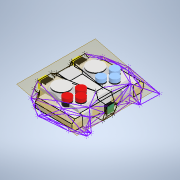
# Autodesk Inventor part: Obudowa_v1_srodek_2d
Saved by Autodesk Inventor 2020 (Build 240168000, 168)
## iProperties
Created: 2020-04-14
Part Number: Obudowa_v1_srodek_2d
Material: Generic
Document SubType Name: Modeling
Designer: atmat
Density: 1 g/cm^3
Appearance: Default
Author: atmat
Autodesk Inventor part; units mm, degrees
ref_plane "XY Plane" through (0, 0, 0) normal (0, 0, 1) x (1, 0, 0)
sketch "Sketch1" plane through (0, 0, 0) normal (0, 1, 0) x (-1, 0, 0)
  line L0 (35.245, 45.085) -> (-35.245, 45.085)
  line L1 (-35.245, 45.085) -> (-35.245, -45.085)
  line L2 (-35.245, -45.085) -> (35.245, -45.085)
  line L3 (35.245, -45.085) -> (35.245, 45.085)
  circle A0 centre (11.745, 29.845) radius 13
  circle A1 centre (11.745, -29.845) radius 13
  line L4 (-10.475, 45.085) -> (-10.475, -45.085) construction
  circle A2 centre (-10.475, 41.905) radius 6.5
  circle A3 centre (-10.475, 17.775) radius 6.5
  circle A4 centre (-10.475, -17.775) radius 6.5
  circle A5 centre (-10.475, -41.905) radius 6.5
  circle A6 centre (-22.545, 29.845) radius 6.5
  circle A7 centre (-22.545, -29.845) radius 6.5
  point P0 (0, 0)
  dimension "d58" = 70.49
  dimension "d0" = 90.17
  dimension "d1" = 45.085
  dimension "d2" = 35.245
  dimension "d3" = 70.49
  dimension "d4" = 15.24
  dimension "d5" = 15.24
  dimension "d6" = 23.5
  dimension "d7" = 23.5
  dimension "d8" = 26
  dimension "d9" = 26
  dimension "d10" = 45.72
  dimension "d11" = 13
  dimension "d12" = 13
  dimension "d13" = 13
  dimension "d14" = 13
  dimension "d15" = 3.18
  dimension "d16" = 3.18
  dimension "d17" = 24.13
  dimension "d18" = 24.13
  dimension "d19" = 13
  dimension "d20" = 12.07
  dimension "d21" = 12.07
  dimension "d22" = 0
  dimension "d23" = 0
  dimension "d24" = 13
  constraints: 10 end point, 8 centre point, 6 point on line, 2 parallel, 2 perpendicular, 1 horizontal
  measures "d0" distance of L2.end L0.start
  measures "d1" distance from line of point (0, 0) L0
  measures "d2" distance from line of point (0, 0) L3
  measures "d3" distance of L1.end L2.end
  measures "d4" distance from line of L0 A0.centre
  measures "d5" distance from line of L2 A1.centre
  measures "d6" distance from line of L3 A1.centre
  measures "d7" distance from line of L3 A0.centre
  measures "d8" diameter of A0
  measures "d9" diameter of A1
  measures "d10" distance between parallel lines of L3 L4
  measures "d11" diameter of A2
  measures "d12" diameter of A3
  measures "d13" diameter of A4
  measures "d14" diameter of A5
  measures "d15" distance from line of L0 A2.centre
  measures "d16" distance from line of L2 A5.centre
  measures "d17" distance of A3.centre A2.centre
  measures "d18" distance of A4.centre A5.centre
  measures "d19" diameter of A6
  measures "d20" horizontal distance of A2.centre A6.centre
  measures "d21" horizontal distance of A5.centre A7.centre
  measures "d22" vertical distance of A6.centre A0.centre
  measures "d23" vertical distance of A7.centre A1.centre
  measures "d24" diameter of A7
extrude "Extrusion1" add sketch "Sketch1" along normal blind 11 contours A0 | A1
sketch "Sketch2" plane through (0, 0, 0) normal (0, 1, 0) x (-1, 0, 0)
  line L0 (35.245, 45.085) -> (-35.245, 45.085)
  line L1 (-35.245, 45.085) -> (-35.245, -45.085)
  line L2 (-35.245, -45.085) -> (35.245, -45.085)
  line L3 (35.245, -45.085) -> (35.245, 45.085)
  circle A0 centre (11.745, 29.845) radius 13
  circle A1 centre (11.745, -29.845) radius 13
  line L4 (-10.475, 45.085) -> (-10.475, -45.085) construction
  circle A2 centre (-10.475, 41.905) radius 6.5
  circle A3 centre (-10.475, 17.775) radius 6.5
  circle A4 centre (-10.475, -17.775) radius 6.5
  circle A5 centre (-10.475, -41.905) radius 6.5
  circle A6 centre (-22.545, 29.845) radius 6.5
  circle A7 centre (-22.545, -29.845) radius 6.5
  point P0 (0, 0)
  dimension "d27" = 90.17
  dimension "d28" = 45.085
  dimension "d29" = 35.245
  dimension "d30" = 70.49
  dimension "d31" = 15.24
  dimension "d32" = 15.24
  dimension "d33" = 23.5
  dimension "d34" = 23.5
  dimension "d35" = 26
  dimension "d36" = 26
  dimension "d37" = 45.72
  dimension "d38" = 13
  dimension "d39" = 13
  dimension "d40" = 13
  dimension "d41" = 13
  dimension "d42" = 3.18
  dimension "d43" = 3.18
  dimension "d44" = 24.13
  dimension "d45" = 24.13
  dimension "d46" = 13
  dimension "d47" = 12.07
  dimension "d48" = 12.07
  dimension "d49" = 0
  dimension "d50" = 0
  dimension "d51" = 13
  constraints: 10 end point, 8 centre point, 6 point on line, 2 parallel, 2 perpendicular, 1 horizontal
  measures "d27" distance of L2.end L0.start
  measures "d28" distance from line of point (0, 0) L0
  measures "d29" distance from line of point (0, 0) L3
  measures "d30" distance of L1.end L2.end
  measures "d31" distance from line of L0 A0.centre
  measures "d32" distance from line of L2 A1.centre
  measures "d33" distance from line of L3 A1.centre
  measures "d34" distance from line of L3 A0.centre
  measures "d35" diameter of A0
  measures "d36" diameter of A1
  measures "d37" distance between parallel lines of L3 L4
  measures "d38" diameter of A2
  measures "d39" diameter of A3
  measures "d40" diameter of A4
  measures "d41" diameter of A5
  measures "d42" distance from line of L0 A2.centre
  measures "d43" distance from line of L2 A5.centre
  measures "d44" distance of A3.centre A2.centre
  measures "d45" distance of A4.centre A5.centre
  measures "d46" diameter of A6
  measures "d47" horizontal distance of A2.centre A6.centre
  measures "d48" horizontal distance of A5.centre A7.centre
  measures "d49" vertical distance of A6.centre A0.centre
  measures "d50" vertical distance of A7.centre A1.centre
  measures "d51" diameter of A7
extrude "Extrusion2" add sketch "Sketch2" along normal blind 7 contours A2 L0 | L0 A2 | A5 L2 | L2 A5 | A3 | A4 | A6 | A7
ref_plane "Work Plane1" through (0, 7, 0) normal (0, 1, 0) x (-1, 0, 0)
sketch "Sketch3" plane through (0, 7, 0) normal (0, 1, 0) x (-1, 0, 0)
  line L0 (35.245, 45.085) -> (-35.245, 45.085)
  line L1 (-35.245, 45.085) -> (-35.245, -45.085)
  line L2 (-35.245, -45.085) -> (35.245, -45.085)
  line L3 (35.245, -45.085) -> (35.245, 45.085)
  circle A0 centre (11.745, 29.845) radius 13
  circle A1 centre (11.745, -29.845) radius 13
  line L4 (-10.475, 45.085) -> (-10.475, -45.085) construction
  circle A2 centre (-10.475, 41.905) radius 6.5
  circle A3 centre (-10.475, 17.775) radius 6.5
  circle A4 centre (-10.475, -17.775) radius 6.5
  circle A5 centre (-10.475, -41.905) radius 6.5
  circle A6 centre (-22.545, 29.845) radius 6.5
  circle A7 centre (-22.545, -29.845) radius 6.5
  point P0 (0, 0)
  dimension "d55" = 90.17
  dimension "d56" = 45.085
  dimension "d57" = 35.245
  dimension "d58" = 70.49
  dimension "d59" = 15.24
  dimension "d60" = 15.24
  dimension "d61" = 23.5
  dimension "d62" = 23.5
  dimension "d63" = 26
  dimension "d64" = 26
  dimension "d65" = 45.72
  dimension "d66" = 13
  dimension "d67" = 13
  dimension "d68" = 13
  dimension "d69" = 13
  dimension "d70" = 3.18
  dimension "d71" = 3.18
  dimension "d72" = 24.13
  dimension "d73" = 24.13
  dimension "d74" = 13
  dimension "d75" = 12.07
  dimension "d76" = 12.07
  dimension "d77" = 0
  dimension "d78" = 0
  dimension "d79" = 13
  constraints: 10 end point, 8 centre point, 6 point on line, 2 parallel, 2 perpendicular, 1 horizontal
  measures "d55" distance of L2.end L0.start
  measures "d56" distance from line of point (0, 0) L0
  measures "d57" distance from line of point (0, 0) L3
  measures "d58" distance of L1.end L2.end
  measures "d59" distance from line of L0 A0.centre
  measures "d60" distance from line of L2 A1.centre
  measures "d61" distance from line of L3 A1.centre
  measures "d62" distance from line of L3 A0.centre
  measures "d63" diameter of A0
  measures "d64" diameter of A1
  measures "d65" distance between parallel lines of L3 L4
  measures "d66" diameter of A2
  measures "d67" diameter of A3
  measures "d68" diameter of A4
  measures "d69" diameter of A5
  measures "d70" distance from line of L0 A2.centre
  measures "d71" distance from line of L2 A5.centre
  measures "d72" distance of A3.centre A2.centre
  measures "d73" distance of A4.centre A5.centre
  measures "d74" diameter of A6
  measures "d75" horizontal distance of A2.centre A6.centre
  measures "d76" horizontal distance of A5.centre A7.centre
  measures "d77" vertical distance of A6.centre A0.centre
  measures "d78" vertical distance of A7.centre A1.centre
  measures "d79" diameter of A7
extrude "Extrusion3" add sketch "Sketch3" along normal blind 6 separate body contours A2 L0 | L0 A2 | A5 L2 | L2 A5 | A3 | A4 | A6 | A7
sketch "Sketch4" plane through (0, 0, 0) normal (0, 1, 0) x (-1, 0, 0)
  line L0 (35.245, 45.085) -> (-35.245, 45.085)
  line L1 (-35.245, 45.085) -> (-35.245, -45.085)
  line L2 (-35.245, -45.085) -> (35.245, -45.085)
  line L3 (35.245, -45.085) -> (35.245, 45.085)
  circle A0 centre (11.745, 29.845) radius 13
  circle A1 centre (11.745, -29.845) radius 13
  line L4 (-10.475, 45.085) -> (-10.475, -45.085) construction
  circle A2 centre (-10.475, 41.905) radius 6.5
  circle A3 centre (-10.475, 17.775) radius 6.5
  circle A4 centre (-10.475, -17.775) radius 6.5
  circle A5 centre (-10.475, -41.905) radius 6.5
  circle A6 centre (-22.545, 29.845) radius 6.5
  circle A7 centre (-22.545, -29.845) radius 6.5
  point P0 (0, 0)
  dimension "d82" = 90.17
  dimension "d83" = 45.085
  dimension "d84" = 35.245
  dimension "d85" = 70.49
  dimension "d86" = 15.24
  dimension "d87" = 15.24
  dimension "d88" = 23.5
  dimension "d89" = 23.5
  dimension "d90" = 26
  dimension "d91" = 26
  dimension "d92" = 45.72
  dimension "d93" = 13
  dimension "d94" = 13
  dimension "d95" = 13
  dimension "d96" = 13
  dimension "d97" = 3.18
  dimension "d98" = 3.18
  dimension "d99" = 24.13
  dimension "d100" = 24.13
  dimension "d101" = 13
  dimension "d102" = 12.07
  dimension "d103" = 12.07
  dimension "d104" = 0
  dimension "d105" = 0
  dimension "d106" = 13
  constraints: 10 end point, 8 centre point, 6 point on line, 2 parallel, 2 perpendicular, 1 horizontal
  measures "d82" distance of L2.end L0.start
  measures "d83" distance from line of point (0, 0) L0
  measures "d84" distance from line of point (0, 0) L3
  measures "d85" distance of L1.end L2.end
  measures "d86" distance from line of L0 A0.centre
  measures "d87" distance from line of L2 A1.centre
  measures "d88" distance from line of L3 A1.centre
  measures "d89" distance from line of L3 A0.centre
  measures "d90" diameter of A0
  measures "d91" diameter of A1
  measures "d92" distance between parallel lines of L3 L4
  measures "d93" diameter of A2
  measures "d94" diameter of A3
  measures "d95" diameter of A4
  measures "d96" diameter of A5
  measures "d97" distance from line of L0 A2.centre
  measures "d98" distance from line of L2 A5.centre
  measures "d99" distance of A3.centre A2.centre
  measures "d100" distance of A4.centre A5.centre
  measures "d101" diameter of A6
  measures "d102" horizontal distance of A2.centre A6.centre
  measures "d103" horizontal distance of A5.centre A7.centre
  measures "d104" vertical distance of A6.centre A0.centre
  measures "d105" vertical distance of A7.centre A1.centre
  measures "d106" diameter of A7
extrude "Extrusion4" add sketch "Sketch4" against normal blind 18 contours L3 L2 A5 L1 L0 A2 | A2 L0 | L2 A5 | A0 | A1 | A3 | A4 | A6 | A7 picked at (-10.0855, 41.5356) picked at (-10.2378, -41.8714) bodies 1
ref_plane "Work Plane2" through (-35.245, 0, 0) normal (1, 0, 0) x (0, 1, 0)
sketch "Sketch6" plane through (-35.245, 0, 0) normal (1, 0, 0) x (0, 1, 0)
  circle A0 centre (0, -29.845) radius 6.5
  circle A1 centre (0, 29.845) radius 6.5
  line L0 (0, -45.085) -> (0, 45.085) projected
  line L1 (6, -23.845) -> (-6, -23.845)
  line L2 (-6, -23.845) -> (-6, -35.845)
  line L3 (-6, -35.845) -> (6, -35.845)
  line L4 (6, -35.845) -> (6, -23.845)
  line L5 (6, 35.845) -> (-6, 35.845)
  line L6 (-6, 35.845) -> (-6, 23.845)
  line L7 (-6, 23.845) -> (6, 23.845)
  line L8 (6, 23.845) -> (6, 35.845)
  point P0 (0, 0)
  dimension "d114" = 13
  dimension "d115" = 13
  dimension "d116" = 59.69
  dimension "d117" = 29.845
  dimension "d149" = 12
  dimension "d150" = 12
  dimension "d151" = 6
  dimension "d152" = 6
  dimension "d153" = 12
  dimension "d154" = 12
  dimension "d155" = 6
  dimension "d156" = 6
  constraints: 16 end point, 4 parallel, 2 centre point, 2 horizontal, 2 perpendicular, 2 point on line
  measures "d114" diameter of A0
  measures "d115" diameter of A1
  measures "d116" distance of A1.centre A0.centre
  measures "d117" distance of point (0, 0) A0.centre
  measures "d149" distance of L5.start L5.end
  measures "d150" distance of L5.end L6.end
  measures "d151" distance from line of A1.centre L5
  measures "d152" distance from line of L6 A1.centre
  measures "d153" distance of L1.start L1.end
  measures "d154" distance of L1.end L2.end
  measures "d155" distance from line of A0.centre L1
  measures "d156" distance from line of A0.centre L2
extrude "Extrusion5" add sketch "Sketch6" against normal blind 7 contours L4 A0 L3 L0 L1 | A0 L1 L4 | L4 L3 A0 | L0 L3 A0 L2 L1 | A0 L2 L1 | L3 L2 A0 | L8 A1 L7 L0 L5 | A1 L5 L8 | L8 L7 A1 | L0 L7 A1 L6 L5 | A1 L6 L5 | L7 L6 A1 bodies 1
ref_plane "Work Plane3" through (-42.245, 0, 0) normal (1, 0, 0) x (0, 1, 0)
sketch "Sketch8" plane through (-35.245, 0, 0) normal (1, 0, 0) x (0, 1, 0)
  circle A0 centre (-9, 54.085) radius 9
  circle A1 centre (-9, -54.085) radius 9
  line L0 (0, 45.085) -> (-18, 45.085) projected
  line L1 (0, -45.085) -> (-18, -45.085) projected
  line L2 (-18, -45.085) -> (-18, 45.085) projected
  line L3 (0, -63.085) -> (-18, -63.085)
  line L4 (-18, -63.085) -> (-18, -45.085)
  line L5 (-18, -45.085) -> (0, -45.085)
  line L6 (0, -45.085) -> (0, -63.085)
  line L7 (0, 45.085) -> (0, -45.085) projected
  line L8 (0, 45.085) -> (-18, 45.085)
  line L9 (-18, 45.085) -> (-18, 63.085)
  line L10 (-18, 63.085) -> (0, 63.085)
  line L11 (0, 63.085) -> (0, 45.085)
  line L12 (-12.7279, -63.085) -> (-18, -57.8129)
  line L13 (-5.2721, -63.085) -> (0, -57.8129)
  line L14 (0, 57.8129) -> (-5.2721, 63.085)
  line L15 (-12.7279, 63.085) -> (-18, 57.8129)
  point P0 (0, 0)
  point P1 (-15.364, 60.449)
  point P2 (-9, 63.085)
  point P3 (-2.636, 60.449)
  point P4 (0, 54.085)
  point P5 (-9, 45.085)
  point P6 (-18, 54.085)
  point P7 (-2.636, -60.449)
  point P8 (-9, -63.085)
  point P9 (-15.364, -60.449)
  point P10 (-18, -54.085)
  point P11 (0, -54.085)
  point P12 (-9, -45.085)
  dimension "d127" = 18
  dimension "d128" = 18
  dimension "d129" = 9
  dimension "d130" = 9
  dimension "d1542" = 45
  dimension "d1543" = 45
  dimension "d1544" = 45
  dimension "d1545" = 45
  constraints: 24 end point, 9 point on line, 9 tangent, 4 parallel, 2 centre point, 2 horizontal, 2 perpendicular
  measures "d127" diameter of A0
  measures "d128" diameter of A1
  measures "d129" horizontal distance of A1.centre point (0, 0)
  measures "d130" horizontal distance of A0.centre point (0, 0)
  measures "d1542" angle of L4 L12
  measures "d1543" angle of L9 L15
  measures "d1544" angle of L10 L14
  measures "d1545" angle of L6 L13
extrude "Extrusion7" add sketch "Sketch8" along normal blind 65 separate body contours A0 | L11 L0 A0 | A0 L14 L11 | A0 L10 L14 | L0 L9 A0 | A0 L15 L10 | L9 L15 A0 | L6 A1 L1 | L1 A1 L4 | A1 | L6 L13 A1 | A1 L12 L4 | L13 L3 A1 | A1 L3 L12
sketch "Sketch9" plane through (0, 7, 0) normal (0, 1, 0) x (-1, 0, 0)
  line L0 (25.245, 13.5) -> (-1.755, 13.5)
  line L1 (-1.755, 13.5) -> (-1.755, -13.5)
  line L2 (-1.755, -13.5) -> (25.245, -13.5)
  line L3 (25.245, -13.5) -> (25.245, 13.5)
  circle A0 centre (11.745, 29.845) radius 13 projected
  circle A1 centre (11.745, 29.845) radius 13
  point P0 (0, 0)
  dimension "d133" = 27
  dimension "d134" = 27
  dimension "d135" = 13.5
  dimension "d136" = 13.5
  constraints: 8 end point, 2 parallel, 1 centre point, 1 coincident, 1 horizontal, 1 perpendicular
  measures "d133" distance of L2.end L0.start
  measures "d134" distance of L1.end L2.end
  measures "d135" distance from line of point (0, 0) L2
  measures "d136" distance from line of L3 A1.centre
sketch "Sketch10" plane through (35.245, 0, 45.085) normal (1, 0, 0) x (0, 0, -1)
  line L0 (40.085, -16) -> (50.085, -16)
  line L1 (50.085, -16) -> (50.085, -6)
  line L2 (50.085, -6) -> (40.085, -6)
  line L3 (40.085, -6) -> (40.085, -16)
  line L4 (0, 0) -> (90.17, 0) projected
  point P0 (45.085, 0)
  dimension "d137" = 10
  dimension "d138" = 10
  dimension "d140" = 5
  dimension "d171" = 6
  constraints: 8 end point, 2 parallel, 1 horizontal, 1 perpendicular
  measures "d137" distance of L1.end L2.end
  measures "d138" distance of L0.end L1.end
  measures "d140" distance from line of point (45.085, 0) L1
  measures "d171" distance between parallel lines of L4 L2
extrude "Extrusion8" add sketch "Sketch10" along normal blind 7 bodies 1
sketch "Sketch11" plane through (42.245, 0, 45.085) normal (1, 0, 0) x (0, 0, -1)
  line L0 (40.085, -16) -> (50.085, -16)
  line L1 (50.085, -16) -> (50.085, -6)
  line L2 (50.085, -6) -> (40.085, -6)
  line L3 (40.085, -6) -> (40.085, -16)
  line L4 (0, 0) -> (90.17, 0) projected
  point P0 (45.085, 0)
  dimension "d143" = 10
  dimension "d144" = 10
  dimension "d146" = 5
  dimension "d172" = 6
  constraints: 8 end point, 2 parallel, 1 horizontal, 1 perpendicular
  measures "d143" distance of L1.end L2.end
  measures "d144" distance of L0.end L1.end
  measures "d146" distance from line of point (45.085, 0) L1
  measures "d172" distance between parallel lines of L4 L2
extrude "Extrusion9" add sketch "Sketch11" along normal blind 3 bodies 1
sketch "Sketch12" plane through (-42.245, 0, 0) normal (1, 0, 0) x (0, 1, 0)
  circle A0 centre (0, -29.845) radius 6.5
  circle A1 centre (0, 29.845) radius 6.5
  line L0 (6, -23.845) -> (-6, -23.845)
  line L1 (-6, -23.845) -> (-6, -35.845)
  line L2 (-6, -35.845) -> (6, -35.845)
  line L3 (6, -35.845) -> (6, -23.845)
  line L4 (6, 35.845) -> (-6, 35.845)
  line L5 (-6, 35.845) -> (-6, 23.845)
  line L6 (-6, 23.845) -> (6, 23.845)
  line L7 (6, 23.845) -> (6, 35.845)
  point P0 (0, 0)
  dimension "d157" = 13
  dimension "d158" = 13
  dimension "d159" = 59.69
  dimension "d160" = 29.845
  dimension "d161" = 12
  dimension "d162" = 12
  dimension "d163" = 6
  dimension "d164" = 6
  dimension "d165" = 12
  dimension "d166" = 12
  dimension "d167" = 6
  dimension "d168" = 6
  constraints: 16 end point, 4 parallel, 2 centre point, 2 horizontal, 2 perpendicular
  measures "d157" diameter of A0
  measures "d158" diameter of A1
  measures "d159" distance of A1.centre A0.centre
  measures "d160" distance of point (0, 0) A0.centre
  measures "d161" distance of L4.start L4.end
  measures "d162" distance of L4.end L5.end
  measures "d163" distance from line of A1.centre L4
  measures "d164" distance from line of L5 A1.centre
  measures "d165" distance of L0.start L0.end
  measures "d166" distance of L0.end L1.end
  measures "d167" distance from line of A0.centre L0
  measures "d168" distance from line of A0.centre L1
extrude "Extrusion10" add sketch "Sketch12" against normal blind 4 separate body contours L3 A0 L2 L1 L0 | A0 L0 L3 | L3 L2 A0 | A0 L1 L0 | L2 L1 A0 | L7 A1 L6 L5 L4 | A1 L4 L7 | L7 L6 A1 | A1 L5 L4 | L6 L5 A1
move faces "Move21" translate (10, 0, 0) faces at (-35.245, -6, -53.5703)
move faces "Move22" translate (10, 0, 0) faces at (-35.245, -6, 53.5703)
move faces "Move23" translate (10, 0, 0) faces at (29.755, -6, 53.5703)
move faces "Move24" translate (10, 0, 0) faces at (29.755, -6, -53.5703)
sketch3d "3D Sketch1"
boundary_patch "Poczatek Wew"
boundary_patch "Boundary Patch173"
boundary_patch "Boundary Patch174"
boundary_patch "Boundary Patch175"
boundary_patch "Boundary Patch176"
boundary_patch "Boundary Patch177"
boundary_patch "Boundary Patch178"
boundary_patch "Boundary Patch179"
boundary_patch "Boundary Patch180"
boundary_patch "Boundary Patch181"
boundary_patch "Boundary Patch182"
boundary_patch "Boundary Patch183"
boundary_patch "Boundary Patch184"
boundary_patch "Boundary Patch185"
boundary_patch "Boundary Patch186"
boundary_patch "Boundary Patch187"
boundary_patch "Boundary Patch188"
boundary_patch "Boundary Patch189"
boundary_patch "Boundary Patch190"
boundary_patch "Boundary Patch191"
thicken "Thicken3" operation add thickness 1 both sides no extend neighbours yes toward (-0.9870503, 0, -0.1604113) bodies 1 faces at (16.1292, 4.6667, -30.8877)
thicken "Thicken4" operation add thickness 1 both sides no extend neighbours yes toward (0.9127874, 0, -0.4084351) bodies 1 faces at (16.4081, 2.3333, -44.5598)
thicken "Thicken5" operation add thickness 1 both sides no extend neighbours yes toward (-0.9870503, 0, -0.1604113) bodies 2 faces at (16.1292, 11, -30.8877)
thicken "Thicken6" operation add thickness 1 both sides no extend neighbours yes toward (-0.9870503, 0, -0.1604113) bodies 2 faces at (4.0592, 11, -18.8177)
thicken "Thicken7" operation add thickness 1 both sides no extend neighbours yes toward (-0.9967573, 0, 0.0804666) bodies 1 faces at (3.9961, 2.3333, -17.252)
thicken "Thicken8" operation add thickness 1 both sides no extend neighbours yes toward (-0.9870503, 0, -0.1604113) bodies 2 faces at (4.0592, 11, -42.9477)
thicken "Thicken9" operation add thickness 1 both sides no extend neighbours yes toward (0.9885186, 0, -0.1510992) bodies 1 faces at (1.1057, 6, -31.8093)
thicken "Thicken10" operation add thickness 1 both sides no extend neighbours yes toward (-0.9870503, 0, -0.1604113) bodies 1 faces at (-24.5767, 7.3333, 27.7597)
thicken "Thicken11" operation add thickness 1 both sides no extend neighbours yes toward (-0.9870503, 0, -0.1604113) bodies 1 faces at (4.0592, 4.6667, 16.7323)
thicken "Thicken12" operation add thickness 1 both sides no extend neighbours yes toward (-0.9870503, 0, -0.1604113) bodies 2 faces at (4.0592, 11, 16.7323)
thicken "Thicken13" operation add thickness 1 both sides no extend neighbours yes toward (-0.9870503, 0, -0.1604113) bodies 1 faces at (16.1292, 4.6667, 28.8023)
thicken "Thicken14" operation add thickness 1 both sides no extend neighbours yes toward (-0.9870503, 0, -0.1604113) bodies 2 faces at (16.1292, 11, 28.8023)
thicken "Thicken15" operation add thickness 1 both sides no extend neighbours yes toward (0.9127874, 0, 0.4084351) bodies 1 faces at (16.4081, 2.3333, 44.5598)
thicken "Thicken16" operation add thickness 1 both sides no extend neighbours yes toward (-0.9870503, 0, -0.1604113) bodies 2 faces at (4.0592, 11, 40.8623)
thicken "Thicken17" operation add thickness 1 both sides no extend neighbours yes toward (0, 1, 0) bodies 1 faces at (-37.5783, 6, 27.845) (-39.9117, 0, 23.845) (-37.5783, -6, 31.845) (-39.9117, 0, 35.845)
thicken "Thicken18" operation add thickness 1 both sides no extend neighbours yes toward (0, 0, -1) bodies 1 faces at (-39.9117, 0, -35.845) (-37.5783, 6, -31.845) (-39.9117, 0, -23.845) (-37.5783, -6, -27.845)
thicken "Thicken19" operation add thickness 1 both sides no extend neighbours yes toward (0, 0, -1) bodies 4 faces at (-43.5783, -2, -35.845) (-43.5783, -6, -27.845) (-43.5783, 6, -31.845) (-43.5783, 2, -23.845)
thicken "Thicken20" operation add thickness 1 both sides no extend neighbours yes toward (0, 0, -1) bodies 4 faces at (-43.5783, -2, 23.845) (-43.5783, 6, 27.845) (-43.5783, 2, 35.845) (-43.5783, -6, 31.845)
thicken "Thicken21" operation add thickness 1 both sides no extend neighbours yes toward (0, 1, 0) bodies 1 faces at (41.9117, -6, 1.6667) (41.9117, -9.3333, -5) (41.9117, -16, 1.6667) (41.9117, -9.3333, 5)
thicken "Thicken22" operation add thickness 3 both sides no extend neighbours yes toward (0, 1, 0) bodies 1 faces at (-30.0626, 0, -6.1077)
boundary_patch "Boundary Patch192"
sketch "Sketch79" plane through (-34.245, 9, 12.5) normal (0.2352941, 0.9719242, 0) x (0.9719242, -0.2352941, 0)
  line L0 (0, 25) -> (0, 0) projected
  line L1 (17, 0) -> (17, 25) projected
  line L2 (0, 25) -> (17, 25)
  line L3 (17, 25) -> (17, 0)
  line L4 (17, 0) -> (0, 0)
  line L5 (0, 0) -> (0, 25)
  point P0 (35.4012, 12.5)
  point P1 (17, 25)
  point P2 (0, 0)
  constraints: 8 end point, 2 parallel, 1 horizontal, 1 perpendicular
extrude "Extrusion76" add sketch "Sketch79" along normal blind 1 and the other way blind 9 bodies 1
move faces "Move26" translate (0, -3, 0) faces at (-13.2754, -18, -2)
sketch "Sketch81" plane through (-35.245, -7, 22.845) normal (-1, 0, 0) x (0, 0, 1)
  line L0 (-27.845, 2) -> (-17.845, 2)
  line L1 (-17.845, 2) -> (-17.845, -10)
  line L2 (-17.845, -10) -> (-27.845, -10)
  line L3 (-27.845, -10) -> (-27.845, 2)
  line L4 (-27.845, 2) -> (-29.845, 0)
  line L5 (-29.845, 0) -> (-29.845, -8)
  line L6 (-29.845, -8) -> (-27.845, -10)
  line L7 (-17.845, -10) -> (-15.845, -8)
  line L8 (-15.845, -8) -> (-15.845, 0)
  line L9 (-15.845, 0) -> (-17.845, 2)
  line L10 (-22.845, 28.6) -> (-22.845, -31.6) projected
  line L11 (-67.93, 7) -> (22.24, 7) projected
  line L12 (-28.845, -11) -> (-16.845, -11)
  line L13 (-16.845, -11) -> (-16.845, -23)
  line L14 (-16.845, -23) -> (-28.845, -23)
  line L15 (-28.845, -23) -> (-28.845, -11)
  line L16 (-27.845, -10) -> (-28.845, -11)
  line L17 (-17.845, -10) -> (-16.845, -11)
  point P0 (-22.845, 7)
  dimension "d1659" = 45
  dimension "d1660" = 45
  dimension "d1661" = 45
  dimension "d1662" = 45
  dimension "d1663" = 10
  dimension "d1664" = 2
  dimension "d1665" = 2
  dimension "d1666" = 5
  dimension "d1667" = 5
  dimension "d1668" = 12
  dimension "d1669" = 30
  dimension "d1670" = 12
  dimension "d1671" = 6
  dimension "d1672" = 12
  constraints: 32 end point, 5 parallel, 2 horizontal, 2 perpendicular, 1 vertical
  measures "d1659" angle of L3 L4
  measures "d1660" angle of L3 L6
  measures "d1661" angle of L1 L7
  measures "d1662" angle of L1 L9
  measures "d1663" distance of L0.start L0.end
  measures "d1664" distance between parallel lines of L3 L5
  measures "d1665" distance between parallel lines of L1 L8
  measures "d1666" distance between parallel lines of L3 L10
  measures "d1667" distance between parallel lines of L11 L0
  measures "d1668" distance between parallel lines of L2 L0
  measures "d1669" distance between parallel lines of L14 L11
  measures "d1670" distance of L13.end L14.end
  measures "d1671" distance between parallel lines of L10 L13
  measures "d1672" distance of L12.end L13.end
extrude "Extrusion78" add sketch "Sketch81" along normal blind 10 and the other way blind 20 bodies 1
move faces "Move27" translate (3, 0, 0) faces at (-35.245, 5.6667, -32.1783)
move faces "Move28" translate (3, 0, 0) faces at (-35.245, 5.6667, 27.5117)
sketch "Sketch82" plane through (39.755, 0, 45.085) normal (0, 0, -1) x (-1, 0, 0)
  line L0 (65, -18) -> (0, -18) projected
  line L1 (0, -18) -> (0, 0) projected
  line L2 (4.51, -18) -> (0, -18)
  line L3 (0, -18) -> (0, 0)
  line L4 (0, 0) -> (4.51, 0)
  line L5 (4.51, 0) -> (4.51, -18)
  line L6 (4.51, 3) -> (4.51, -21) projected
  point P0 (39.755, 0)
  dimension "d1683" = 0
  constraints: 8 end point, 2 parallel, 1 horizontal, 1 perpendicular, 1 point on line
  measures "d1683" distance between parallel lines of L6 L5
extrude "Extrusion79" add sketch "Sketch82" along normal blind 18 separate body
sketch "Sketch83" plane through (35.245, -18, -45.085) normal (0, 0, 1) x (1, 0, 0)
  line L0 (4.51, 18) -> (4.51, 0) projected
  line L1 (0, 18) -> (0, 0) projected
  line L2 (4.51, 18) -> (0, 18)
  line L3 (0, 18) -> (0, 0)
  line L4 (0, 0) -> (4.51, 0)
  line L5 (4.51, 0) -> (4.51, 18)
  point P0 (-35.245, 18)
  constraints: 8 end point, 2 parallel, 1 horizontal, 1 perpendicular
extrude "Extrusion80" add sketch "Sketch83" along normal blind 18 separate body
thicken "Thicken23" operation add thickness 2 both sides no extend neighbours no toward (0, 1, 0) bodies 1 faces at (33.439, 3, 9.35)
chamfer "Chamfer1" distance 4 angle 45 1 edges at (35.245, 5, 0)
chamfer "Chamfer2" distance 4 angle 45 10 edges at (35.245, -11, 6) (35.245, -11, -6) (-35.245, -1, -22.845) (-35.245, -1, 22.845) (-35.245, -1, 36.845) (-35.245, -1, -36.845) (-35.245, -7, -29.845) (-35.245, -7, 29.845) (35.245, -17, 0) (35.245, -5, 0)
chamfer "Chamfer3" distance 4 angle 45 2 edges at (2.255, 5, 29.845) (2.255, 5, -29.845)
ref_plane "Work Plane11" through (-34.245, 9, -12.5) normal (0.2352941, 0.9719242, 0) x (0, 0, 1)
sketch "Sketch84" plane through (-34.245, 9, -12.5) normal (0.2352941, 0.9719242, 0) x (0, 0, 1)
  line L0 (26, 0) -> (-1, 0)
  line L1 (-1, 0) -> (-1, 18)
  line L2 (-1, 18) -> (26, 18)
  line L3 (26, 18) -> (26, 0)
  line L4 (0, 17) -> (0, 0) projected
  line L5 (0, 0) -> (25, 0) projected
  line L6 (25, 0) -> (25, 17) projected
  line L7 (25, 17) -> (0, 17)
  line L8 (0, 17) -> (0, 0)
  line L9 (0, 0) -> (25, 0)
  line L10 (25, 0) -> (25, 17)
  point P0 (12.5, 35.4012)
  point P1 (25, 0)
  dimension "d1699" = 1
  dimension "d1700" = 0
  dimension "d1701" = 1
  dimension "d1702" = 1
  constraints: 16 end point, 3 parallel, 3 perpendicular, 2 horizontal
  measures "d1699" distance between parallel lines of L4 L1
  measures "d1700" distance between parallel lines of L5 L0
  measures "d1701" distance between parallel lines of L7 L2
  measures "d1702" distance between parallel lines of L10 L3
extrude "Extrusion81" add sketch "Sketch84" against normal blind 9 contours L0 L6 L7 L4 L1 L2 L3 bodies 1
sketch "Sketch85" plane through (17.2675, 5, 45.085) normal (0, 1, 0) x (1, 0, 0)
  line L0 (-17.2675, 59.085) -> (-57.2675, 59.085)
  line L1 (-57.2675, 59.085) -> (-57.2675, 31.085)
  line L2 (-57.2675, 31.085) -> (-17.2675, 31.085)
  line L3 (-17.2675, 31.085) -> (-17.2675, 59.085)
  point P0 (-17.2675, 45.085)
  dimension "d1705" = 40
  dimension "d1706" = 28
  dimension "d1707" = 14
  dimension "d1708" = 0
  constraints: 8 end point, 2 parallel, 1 horizontal, 1 perpendicular
  measures "d1705" distance of L1.end L2.end
  measures "d1706" distance of L2.end L0.start
  measures "d1707" distance from line of point (-17.267, 45.085) L2
  measures "d1708" distance from line of point (-17.267, 45.085) L3
extrude "Extrusion82" add sketch "Sketch85" against normal blind 5 bodies 1
chamfer "Chamfer5" distance 2 angle 45 1 edges at (-40, 5, 0)
body "Solid1"
body "Solid2"
body "Solid5"
body "Solid6"
body "Srf172"
body "Srf173"
body "Srf174"
body "Srf175"
body "Srf176"
body "Srf177"
body "Srf178"
body "Srf179"
body "Srf180"
body "Srf181"
body "Srf182"
body "Srf183"
body "Srf184"
body "Srf185"
body "Srf186"
body "Srf187"
body "Srf188"
body "Srf189"
body "Srf190"
body "Srf191"
body "Srf192"
body "Solid9"
body "Solid10"
